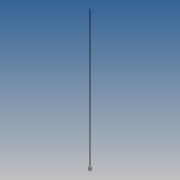
# Autodesk Inventor part: 2f3lna
Saved by Autodesk Inventor 2014 SP1 (Build 180222100, 222)
## iProperties
Company: HERA Project
Created: 2013-06-04
Part Number: 2f3lna
Material: Aluminum 6061
Document SubType Name: Modeling
Designer: David DeBoer
Density: 2.71 g/cm^3
Description: Feed lna dummy load
Mass: 757.978 g
Surface Area: 501.749 cm^2
Volume: 279.697 cm^3
Appearance: Aluminum - Flat
Author: David DeBoer
Title: Feed dummy lna
Autodesk Inventor part; units mm, degrees
ref_plane "YZ Plane" through (0, 0, 0) normal (1, 0, 0) x (0, 1, 0)
ref_plane "XZ Plane" through (0, 0, 0) normal (0, 1, 0) x (-1, 0, 0)
ref_plane "XY Plane" through (0, 0, 0) normal (0, 0, 1) x (1, 0, 0)
sketch "Sketch1" plane through (0, 0, 0) normal (0, 1, 0) x (-1, 0, 0)
  circle A0 centre (0, 0) radius 9.525
  circle A1 centre (0, 0) radius 6.985
  dimension "d0" = 19.05
  dimension "d2" = 2.54
  constraints: 2 centre point, 1 coincident
  measures "d0" diameter of A0
  measures "d2" radial gap between concentric circles of A1 A0
extrude "Extrusion1" add sketch "Sketch1" along normal blind 101.6
sketch "Sketch2" plane through (0, 101.6, 0) normal (0, 1, 0) x (1, 0, 0)
  circle A0 centre (0, 0) radius 9.525 projected
  line L0 (-9.525, 0) -> (-34.925, 0)
  line L1 (-34.925, 0) -> (-34.925, 25.4)
  line L2 (-34.925, 25.4) -> (-9.525, 25.4)
  line L3 (-9.525, 25.4) -> (-9.525, 0)
  line L4 (-34.925, 0) -> (-34.925, -25.4)
  line L5 (-34.925, -25.4) -> (-9.525, -25.4)
  line L6 (-9.525, -25.4) -> (-9.525, 0)
  line L7 (0, 0) -> (0, -23.8632) construction
  line L8 (9.525, 0) -> (34.925, 0)
  line L9 (34.925, 0) -> (34.925, 25.4)
  line L10 (34.925, 25.4) -> (9.525, 25.4)
  line L11 (9.525, 25.4) -> (9.525, 0)
  line L12 (34.925, 0) -> (34.925, -25.4)
  line L13 (34.925, -25.4) -> (9.525, -25.4)
  line L14 (9.525, -25.4) -> (9.525, 0)
  dimension "d7" = 25.4
  dimension "d17" = 25.4
  constraints: 30 end point, 8 symmetric about line, 3 parallel, 1 horizontal, 1 horizontal alignment, 1 perpendicular, 1 other
  measures "d7" distance of L0.end L1.end
  measures "d17" distance of L4.end L5.end
extrude "Extrusion2" add sketch "Sketch2" against normal blind 101.6 contours L6 L5 L4 L0 | L0 L1 L2 L3 | L11 L10 L9 L8 | L8 L12 L13 L14
sketch "Sketch3" plane through (0, 101.6, 0) normal (0, 1, 0) x (1, 0, 0)
  circle A0 centre (-22.225, 0) radius 2.54
  circle A1 centre (22.225, 0) radius 2.54
  line L0 (9.525, 25.4) -> (9.525, 0) projected
  line L1 (-9.525, 0) -> (-9.525, 25.4) projected
  point P0 (0, 0)
  dimension "d11" = 5.08
  dimension "d12" = 5.08
  dimension "d15" = 12.7
  dimension "d16" = 12.7
  constraints: 2 centre point
  measures "d11" diameter of A0
  measures "d12" diameter of A1
  measures "d15" distance from line of L1 A0.centre
  measures "d16" distance from line of L0 A1.centre
extrude "Extrusion3" add sketch "Sketch3" along normal blind 4064
sketch "Sketch4" plane through (0, 0, 0) normal (0, -1, 0) x (1, 0, 0)
  line L0 (-34.925, -25.4) -> (-9.525, -25.4) projected
  circle A0 centre (-22.225, 12.7) radius 5.08
  circle A1 centre (-22.225, -12.7) radius 5.08
  line L1 (0, 0) -> (0, 23.8246) construction
  circle A2 centre (22.225, 12.7) radius 5.08
  circle A3 centre (22.225, -12.7) radius 5.08
  dimension "d18" = 10.16
  dimension "d19" = 10.16
  constraints: 4 centre point, 2 end point, 2 symmetric about line, 1 perpendicular, 2 other
  measures "d18" diameter of A0
  measures "d19" diameter of A1
extrude "Extrusion4" add sketch "Sketch4" along normal blind 12.7
body "Solid1"
